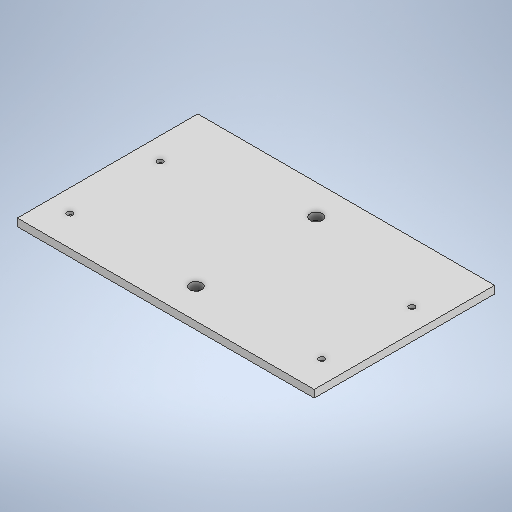
# Autodesk Inventor part: panel2
Saved by Autodesk Inventor 2025.3 (Build 293356000, 356)
## iProperties
Created: 2026-04-19
Part Number: panel2
Material: Generic
Document SubType Name: Modeling
Designer: ksawe
Density: 1 g/cm^3
Appearance: Default
Author: ksawe
Autodesk Inventor part; units mm, degrees
ref_plane "YZ Plane" through (0, 0, 0) normal (1, 0, 0) x (0, 1, 0)
ref_plane "XZ Plane" through (0, 0, 0) normal (0, 1, 0) x (-1, 0, 0)
ref_plane "XY Plane" through (0, 0, 0) normal (0, 0, 1) x (1, 0, 0)
sketch "Sketch1" plane through (0, 0, 0) normal (0, 1, 0) x (-1, 0, 0)
  line L0 (98.75, 60) -> (-98.75, 60)
  line L1 (-98.75, 60) -> (-98.75, -60)
  line L2 (-98.75, -60) -> (98.75, -60)
  line L3 (98.75, -60) -> (98.75, 60)
  line L4 (98.75, 60) -> (-98.75, -60) construction
  line L5 (-98.75, 60) -> (98.75, -60) construction
  circle A0 centre (0, -40) radius 4
  circle A1 centre (0, 40) radius 4
  point P0 (0, 0)
  dimension "d0" = 197.5
  dimension "d1" = 120
  dimension "d2" = 8
  dimension "d3" = 20
  dimension "d4" = 8
  dimension "d5" = 80
  constraints: 12 end point, 2 centre point, 2 midpoint, 2 parallel, 2 vertical alignment, 1 horizontal, 1 perpendicular
  measures "d0" distance of L2.end L1.end
  measures "d1" distance of L0.end L1.end
  measures "d2" diameter of A0
  measures "d3" distance from line of L2 A0.centre
  measures "d4" diameter of A1
  measures "d5" distance of A0.centre A1.centre
extrude "Extrusion1" add sketch "Sketch1" along normal blind 5
sketch "Sketch2" plane through (0, 5, 0) normal (0, 1, 0) x (1, 0, 0)
  line L0 (-98.75, 60) -> (-98.75, -60) projected
  line L1 (98.75, -60) -> (98.75, 60) projected
  line L2 (98.75, 60) -> (-98.75, 60) projected
  line L3 (-98.75, -60) -> (98.75, -60) projected
  point P0 (0, 0)
  point P1 (-83.75, 20)
  point P2 (-83.75, -40)
  point P3 (83.75, -40)
  point P4 (83.75, 20)
  dimension "d8" = 15
  dimension "d9" = 15
  dimension "d17" = 15
  dimension "d18" = 15
  dimension "d19" = 40
  dimension "d20" = 40
  dimension "d21" = 20
  dimension "d22" = 20
  measures "d8" distance from line of L0 point (-83.75, -40)
  measures "d9" distance from line of L0 point (-83.75, 20)
  measures "d17" distance from line of L1 point (83.75, -40)
  measures "d18" distance from line of L1 point (83.75, 20)
  measures "d19" distance from line of L2 point (83.75, 20)
  measures "d20" distance from line of L2 point (-83.75, 20)
  measures "d21" distance from line of L3 point (-83.75, -40)
  measures "d22" distance from line of L3 point (83.75, -40)
hole "Hole1" at (83.75, 5, -20) at (-83.75, 5, -20) at (-83.75, 5, 40) at (83.75, 5, 40) direction (0, -1, 0) diameter 2 depth 4 tip angle 118 counterbore diameter 3.9 counterbore depth 2
body "Solid1"
